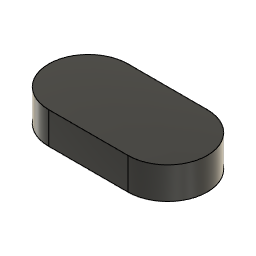
Shock_Pad (Autodesk Fusion 360 design; units mm, degrees)
Autodesk Fusion 360 part; units mm, degrees
sketch "草图1" plane through (0, 0, 0) normal (0, 0, 1) x (1, 0, 0)
  line L0 (-15, -21.6392) -> (0, -21.6392)
  arc A0 (0, -21.6392) -> (0, -6.6392) centre (0, -14.1392) ccw
  line L1 (0, -6.6392) -> (-15, -6.6392)
  arc A1 (-15, -6.6392) -> (-15, -21.6392) centre (-15, -14.1392) ccw
  line L2 (-15, -14.1392) -> (0, -14.1392) construction
  dimension "d1" = 15
  dimension "d2" = 15
  constraint tangent L0 A0
  constraint tangent A0 L1
  constraint parallel L0 L1
  constraint tangent L1 A1
  constraint tangent L0 A1
  constraint horizontal L2
  measures "d1" distance of L0 L1
  measures "d2" distance of A1.centre A0.centre
extrude "拉伸1" add sketch "草图1" along normal blind 6
